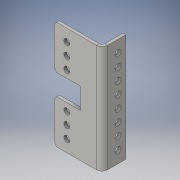
# Autodesk Inventor part: Transmission bracket
Saved by Autodesk Inventor 2016 SP2 (Build 200236200, 236)
## iProperties
Created: 2018-01-18
Part Number: Transmission bracket
Material: Generic
Document SubType Name: Sheet Metal
Designer: CAD
Density: 1 g/cm^3
Sheet Metal Rule: Default
Appearance: Default
Author: CAD
Autodesk Inventor part; units mm, degrees
ref_plane "YZ Plane" through (0, 0, 0) normal (1, 0, 0) x (0, 1, 0)
ref_plane "XZ Plane" through (0, 0, 0) normal (0, 1, 0) x (-1, 0, 0)
ref_plane "XY Plane" through (0, 0, 0) normal (0, 0, 1) x (1, 0, 0)
sketch "Sketch1" plane through (0, 0, 0) normal (0, 0, 1) x (1, 0, 0)
  line L0 (0, 46.0375) -> (-2.644, 42.0764)
  line L1 (-2.644, 42.0764) -> (-2.644, 3.9764)
  line L2 (-2.644, 3.9764) -> (0, 0)
  line L3 (0, 46.0375) -> (25.4, 46.0375)
  line L4 (25.4, 46.0375) -> (25.4, 68.2625)
  line L5 (25.4, 57.15) -> (26.8908, 57.15)
  line L6 (0, 68.2625) -> (-2.644, 72.2236)
  line L7 (-2.644, 72.2236) -> (-2.644, 110.3236)
  line L8 (-2.644, 110.3236) -> (0, 114.3)
  line L9 (0, 68.2625) -> (25.4, 68.2625)
  line L10 (25.4, 68.2625) -> (25.4, 46.0375)
  line L11 (48.156, 114.3) -> (0, 114.3)
  line L12 (48.156, 114.3) -> (48.156, 0)
  line L13 (0, 0) -> (48.156, 0)
  line L14 (218.3648, 132.2525) -> (215.7208, 128.2914)
  line L15 (215.7208, 128.2914) -> (215.7208, 90.1914)
  line L16 (215.7208, 90.1914) -> (218.3648, 86.215)
  line L17 (218.3648, 132.2525) -> (234.2398, 132.2525)
  line L18 (218.3648, 154.4775) -> (215.7208, 158.4387)
  line L19 (215.7208, 158.4387) -> (215.7208, 196.5387)
  line L20 (215.7208, 196.5387) -> (218.3648, 200.515)
  line L21 (218.3648, 154.4775) -> (234.2398, 154.4775)
  line L22 (253.8208, 200.515) -> (218.3648, 200.515)
  line L23 (253.8208, 200.515) -> (253.8208, 86.215)
  line L24 (218.3648, 86.215) -> (253.8208, 86.215)
  line L25 (379.0105, 160.3375) -> (376.3665, 156.3764)
  line L26 (376.3665, 156.3764) -> (376.3665, 118.2764)
  line L27 (376.3665, 118.2764) -> (379.0105, 114.3)
  line L28 (379.0105, 160.3375) -> (398.0605, 160.3375)
  line L29 (398.0605, 160.3375) -> (398.0605, 182.5625)
  line L30 (398.0605, 171.45) -> (393.2013, 171.45)
  line L31 (379.0105, 182.5625) -> (376.3665, 186.5236)
  line L32 (376.3665, 186.5236) -> (376.3665, 224.6236)
  line L33 (376.3665, 224.6236) -> (379.0105, 228.6)
  line L34 (379.0105, 182.5625) -> (398.0605, 182.5625)
  line L35 (398.0605, 182.5625) -> (398.0605, 160.3375)
  line L36 (414.4665, 228.6) -> (379.0105, 228.6)
  line L37 (414.4665, 228.6) -> (414.4665, 114.3)
  line L38 (379.0105, 114.3) -> (414.4665, 114.3)
  line L39 (237.4148, 151.3025) -> (237.4148, 135.4275)
  arc A0 (237.4148, 151.3025) -> (234.2398, 154.4775) centre (234.2398, 151.3025) ccw
  arc A1 (234.2398, 132.2525) -> (237.4148, 135.4275) centre (234.2398, 135.4275) ccw
  line L40 (0, 114.3) -> (48.156, 114.3)
  line L41 (48.156, 114.3) -> (48.156, 0)
  line L42 (48.156, 0) -> (0, 0)
  line L43 (0, 0) -> (-2.644, 3.9764)
  line L44 (-2.644, 3.9764) -> (-2.644, 42.0764)
  line L45 (-2.644, 42.0764) -> (0, 46.0375)
  line L46 (0, 46.0375) -> (25.4, 46.0375)
  line L47 (25.4, 46.0375) -> (25.4, 68.2625)
  line L48 (25.4, 68.2625) -> (0, 68.2625)
  line L49 (0, 68.2625) -> (-2.644, 72.2236)
  line L50 (-2.644, 72.2236) -> (-2.644, 110.3236)
  line L51 (-2.644, 110.3236) -> (0, 114.3)
  dimension "d1" = 46.0375
  dimension "d5" = 38.1
  dimension "d6" = 4.7625
  dimension "d8" = 4.7752
  dimension "d9" = 25.4
  dimension "d12" = 22.225
  dimension "d14" = 114.3
  dimension "d15" = 22.756
  dimension "d16" = 21.2652
  dimension "d26" = 46.0375
  dimension "d27" = 38.1
  dimension "d28" = 4.7625
  dimension "d29" = 4.7752
  dimension "d30" = 19.05
  dimension "d31" = 22.225
  dimension "d32" = 114.3
  dimension "d33" = 16.406
  dimension "d34" = 21.2652
  dimension "d35" = 3.175
  measures "d1" distance of L2.end L0.start
  measures "d5" distance of L0.end L1.end
  measures "d6" distance of L0.start L0.end
  measures "d8" distance of L1.end L2.end
  measures "d9" distance of L0.start L3.end
  measures "d12" distance of L3.end L4.end
  measures "d14" distance of L11.start L12.end
  measures "d15" distance between parallel lines of L12 L4
  measures "d16" distance from line of L5.end L12
  measures "d26" distance of L38.start L28.start
  measures "d27" distance of L25.end L26.end
  measures "d28" distance of L28.start L25.end
  measures "d29" distance of L26.end L38.start
  measures "d30" distance of L28.start L29.start
  measures "d31" distance of L29.start L29.end
  measures "d32" distance of L37.start L37.end
  measures "d33" distance between parallel lines of L37 L29
  measures "d34" distance from line of L30.end L37
  measures "d35" radius of A0
extrude "Plate1" add sketch "Sketch1" along normal blind 3.048 contours L3 L4 L9 L6 L7 L8 L11 L12 L13 L2 L1 L0
sketch "Sketch5" plane through (45.108, 0, 3.048) normal (1, 0, 0) x (0, 1, 0)
  line L0 (114.3, 0) -> (0, 0)
  line L1 (0, 0) -> (0, -25.4)
  line L2 (0, -25.4) -> (114.3, -25.4)
  line L3 (114.3, -25.4) -> (114.3, 0)
  constraints: 6 end point, 1 horizontal, 1 perpendicular, 1 vertical
edge flange "Flange1" height 25.4 angle 90 thickness 3.048 bend radius 3.048 thickness toward (1, 0, 0) relief tear relief width 3.048 relief depth 1.524 edges at (48.156, 57.15, 0) wall of the first edge with corners at (45.108, 114.3, 3.048) (45.108, 0, 3.048) (45.108, 0, -22.352) (45.108, 114.3, -22.352)
bend "Bend2"
corner "Corner1"
sketch "Sketch6" plane through (0, 0, 0) normal (0, 0, -1) x (-1, 0, 0)
  line L0 (0, 114.3) -> (-42.06, 114.3) projected
  line L1 (0, 0) -> (-42.06, 0) projected
  point P0 (-10.9909, 101.6)
  point P1 (-10.9909, 88.9)
  point P2 (-10.9909, 76.2)
  point P3 (-10.9909, 38.1)
  point P4 (-10.9909, 25.4)
  point P5 (-10.9909, 12.7)
  dimension "d91" = 12.7
  dimension "d92" = 12.7
  dimension "d93" = 12.7
  dimension "d94" = 12.7
  dimension "d95" = 12.7
  dimension "d96" = 12.7
  measures "d91" distance from line of L0 point (-10.991, 101.6)
  measures "d92" distance of point (-10.991, 101.6) point (-10.991, 88.9)
  measures "d93" distance of point (-10.991, 88.9) point (-10.991, 76.2)
  measures "d94" distance from line of L1 point (-10.991, 12.7)
  measures "d95" distance of point (-10.991, 25.4) point (-10.991, 12.7)
  measures "d96" distance of point (-10.991, 38.1) point (-10.991, 25.4)
hole "Hole3" at (10.9909, 101.6, 0) at (10.9909, 88.9, 0) at (10.9909, 76.2, 0) at (10.9909, 38.1, 0) at (10.9909, 25.4, 0) at (10.9909, 12.7, 0) direction (0, 0, 1) diameter 6.35 depth 3.048 tip angle 118
sketch "Sketch7" plane through (48.156, 0, -22.352) normal (1, 0, 0) x (0, 0, -1)
  line L0 (0, 0) -> (-19.304, 0) projected
  point P0 (-22.352, 0)
  point P1 (-8.5162, 101.6)
  point P2 (-8.5162, 88.9)
  point P3 (-8.5162, 76.2)
  point P4 (-8.5162, 63.5)
  point P5 (-8.5162, 50.8)
  point P6 (-8.5162, 38.1)
  point P7 (-8.5162, 25.4)
  point P8 (-8.5162, 12.7)
  dimension "d104" = 12.7
  dimension "d105" = 12.7
  dimension "d106" = 12.7
  dimension "d107" = 12.7
  dimension "d108" = 12.7
  dimension "d109" = 12.7
  dimension "d110" = 12.7
  dimension "d111" = 12.7
  measures "d104" distance from line of L0 point (-8.516, 12.7)
  measures "d105" distance of point (-8.516, 12.7) point (-8.516, 25.4)
  measures "d106" distance of point (-8.516, 25.4) point (-8.516, 38.1)
  measures "d107" distance of point (-8.516, 38.1) point (-8.516, 50.8)
  measures "d108" distance of point (-8.516, 50.8) point (-8.516, 63.5)
  measures "d109" distance of point (-8.516, 63.5) point (-8.516, 76.2)
  measures "d110" distance of point (-8.516, 76.2) point (-8.516, 88.9)
  measures "d111" distance of point (-8.516, 88.9) point (-8.516, 101.6)
hole "Hole4" at (48.156, 88.9, -13.8358) at (48.156, 101.6, -13.8358) at (48.156, 76.2, -13.8358) at (48.156, 63.5, -13.8358) at (48.156, 50.8, -13.8358) at (48.156, 25.4, -13.8358) at (48.156, 38.1, -13.8358) at (48.156, 12.7, -13.8358) direction (-1, 0, 0) diameter 6.35 depth 3.048 tip angle 118
equation "\"d92\" = d91"
equation "\"d93\" = d91"
equation "\"d94\" = d91"
equation "\"d95\" = d91"
equation "\"d96\" = d91"
equation "\"d102\" = Thickness"
equation "\"d105\" = d104"
equation "\"d106\" = d104"
equation "\"d107\" = d104"
equation "\"d108\" = d104"
equation "\"d109\" = d104"
equation "\"d110\" = d104"
equation "\"d111\" = d104"
equation "\"d117\" = Thickness"
equation "\"d81\" = BendReliefWidth"
equation "\"d82\" = BendReliefDepth"
equation "\"d83\" = MinimumRemnant"
equation "\"d84\" = BendRadius"
equation "\"d87\" = BendRadius"
equation "\"d88\" = CornerReliefSize"
equation "\"d89\" = GapSize"
equation "\"d90\" = JacobiRadiusSize"
equation "\"BendRadius\" = Thickness"
equation "\"BendReliefWidth\" = Thickness"
equation "\"BendReliefDepth\" = 0.5 * Thickness"
equation "\"CornerReliefSize\" = 4 * Thickness"
equation "\"MinimumRemnant\" = 2 * Thickness"
equation "\"TransitionRadius\" = BendRadius"
equation "\"JacobiRadiusSize\" = BendRadius"
equation "\"GapSize\" = Thickness"
equation "\"d36\" = BendRadius"
equation "\"Thickness\" = 3.048"
body "Solid1"
